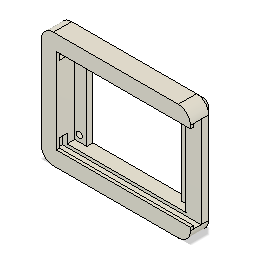
Displaygehäuse (Autodesk Fusion 360 design; units mm, degrees)
Autodesk Fusion 360 part; units mm, degrees
sketch "Skizze1" plane through (0, 0, 0) normal (0, 0, 1) x (1, 0, 0)
  line L0 (19.5, 14) -> (-19.5, 14)
  line L1 (-19.5, 14) -> (-19.5, -14)
  line L2 (-19.5, -14) -> (19.5, -14)
  line L3 (19.5, -14) -> (19.5, 14)
  line L4 (19.5, 14) -> (-19.5, -14) construction
  line L5 (-19.5, 14) -> (19.5, -14) construction
  line L6 (22.5, 17) -> (-22.5, 17)
  line L7 (-22.5, 17) -> (-22.5, -17)
  line L8 (-22.5, -17) -> (22.5, -17)
  line L9 (22.5, -17) -> (22.5, 17)
  line L10 (22.5, 17) -> (-22.5, -17) construction
  line L11 (-22.5, 17) -> (22.5, -17) construction
  line L12 (15.5, 14) -> (-15.5, 14)
  line L13 (-15.5, 14) -> (-15.5, -14)
  line L14 (-15.5, -14) -> (15.5, -14)
  line L15 (15.5, -14) -> (15.5, 14)
  line L16 (15.5, 14) -> (-15.5, -14) construction
  line L17 (-15.5, 14) -> (15.5, -14) construction
  line L18 (-19.5, 14) -> (-18.5, 14)
  circle A0 centre (-18, 12) radius 1
  circle A1 centre (-18, -12) radius 1
  circle A2 centre (18, -12) radius 1
  circle A3 centre (18, 12) radius 1
  dimension "d1" = 39
  dimension "d2" = 28
  dimension "d3" = 45
  dimension "d4" = 34
  dimension "d5" = 31
  dimension "d7" = 2
  dimension "d8" = 2
  dimension "d9" = 2
  dimension "d10" = 2
  constraint horizontal L0
  constraint perpendicular L0 L1
  constraint parallel L0 L2
  constraint parallel L1 L3
  constraint coincident L4 origin
  constraint coincident L5 origin
  constraint horizontal L6
  constraint perpendicular L6 L7
  constraint parallel L6 L8
  constraint parallel L7 L9
  constraint coincident L10 origin
  constraint coincident L11 origin
  constraint horizontal L12
  constraint perpendicular L12 L13
  constraint parallel L12 L14
  constraint parallel L13 L15
  constraint coincident L16 origin
  constraint coincident L17 origin
  constraint coincident L0 L18.end
  measures "d1" distance of L1.end L2.end
  measures "d2" distance of L0.end L1.end
  measures "d3" distance of L7.end L8.end
  measures "d4" distance of L6.start L8.end
  measures "d5" distance of L13.end L14.end
  measures "d7" diameter of A1
  measures "d8" diameter of A0
  measures "d9" diameter of A2
  measures "d10" diameter of A3
extrude "Extrusion1" add sketch "Skizze1" along normal blind 6 contours L6 L7 L8 L9
extrude "Extrusion2" add sketch "Skizze1" along normal blind 2 contours L0 L2 L3 L15 | L0 L1 L2 L13 L18
extrude "Extrusion3" add 1 faces at (-6.5, -16, 6) along direction (0, 0, 1) blind 2
extrude "Extrusion4" add 1 faces at (-22.5, -5.6667, 5.3333) along direction (-1, 0, 0) blind 2
extrude "Extrusion5" add 1 faces at (22.5, -5.6667, 2.6667) along direction (1, 0, 0) blind 2
extrude "Extrusion6" add 1 faces at (-8.1667, -17, 5.3333) along direction (0, -1, 0) blind 2
extrude "Extrusion7" add 1 faces at (8.1667, 17, 5.3333) along direction (0, 1, 0) blind 2
fillet "Abrundung1" radius 4 1 edges at (24.5, 19, 4)
fillet "Abrundung2" radius 4 1 edges at (-24.5, 19, 4)
fillet "Abrundung3" radius 4 1 edges at (-24.5, -19, 4)
fillet "Abrundung4" radius 4 1 edges at (24.5, -19, 4)
chamfer "Fase1" distance 2 angle 45 8 edges at (24.5, 0, 0) (23.3284, -17.8284, 0) (0, -19, 0) (-23.3284, -17.8284, 0) (-24.5, 0, 0) (-23.3284, 17.8284, 0) (0, 19, 0) (23.3284, 17.8284, 0)
sketch "Skizze2" plane through (24.5, 0, 0) normal (1, 0, 0) x (0, 0, -1)
  line L0 (-2, -15) -> (-2, 15)
  line L1 (-2, 15) -> (-8, 15)
  line L2 (-8, 15) -> (-8, -15)
  line L3 (-8, -15) -> (-2, -15)
  line L4 (-7, 15) -> (-4.5, 15)
  line L5 (-4.5, 15) -> (-4.5, -15)
  line L6 (-4.5, -15) -> (-7, -15)
  line L7 (-7, -15) -> (-7, 15)
  constraint horizontal L4
  constraint vertical L5
  constraint horizontal L6
  constraint vertical L7
  constraint coincident L3 L5.end
  constraint coincident L1 L4.start
extrude "Extrusion8" cut sketch "Skizze2" against normal blind 44 contours L1 L3 L4 L5 L6 L7
sketch "Skizze3" plane through (0, 0, 0) normal (1, 0, 0) x (0, 0, -1)
  line L0 (-4.5, -14) -> (-2, -14)
  line L1 (-2, -14) -> (-2, 14)
  line L2 (-2, 14) -> (-4.5, 14)
  line L3 (-4.5, 14) -> (-4.5, 15)
  line L4 (-4.5, 15) -> (-7, 15)
  line L5 (-7, 15) -> (-7, 14)
  line L6 (-7, 14) -> (-8, 14)
  line L7 (-8, 14) -> (-8, -14)
  line L8 (-8, -14) -> (-7, -14)
  line L9 (-7, -14) -> (-7, -15)
  line L10 (-7, -15) -> (-4.5, -15)
  line L11 (-4.5, -15) -> (-4.5, -14)
  line L12 (-7, 15) -> (-4.5, 15)
  line L13 (-4.5, 15) -> (-4.5, 11)
  line L14 (-4.5, 11) -> (-7, 11)
  line L15 (-7, 11) -> (-7, 15)
  line L16 (-7, -15) -> (-4.5, -15)
  line L17 (-4.5, -15) -> (-4.5, -11)
  line L18 (-4.5, -11) -> (-7, -11)
  line L19 (-7, -11) -> (-7, -15)
  dimension "d37" = 4
  dimension "d38" = 2.5
  dimension "d39" = 4
  dimension "d40" = 2.5
  constraint horizontal L12
  constraint vertical L13
  constraint horizontal L14
  constraint vertical L15
  constraint coincident L4.end L5.start
  constraint horizontal L16
  constraint vertical L17
  constraint horizontal L18
  constraint vertical L19
  constraint coincident L9.end L10.start
  measures "d37" distance of L4.end L14.end
  measures "d38" distance of L4.end L3.end
  measures "d39" distance of L9.end L18.end
  measures "d40" distance of L9.end L10.end
extrude "Extrusion9" cut sketch "Skizze3" against normal blind 21 contours L9 L10 L11 L16 L17 L18 L19 | L3 L4 L5 L12 L13 L14 L15
sketch "Skizze4" plane through (19.5, 0, 0) normal (-1, 0, 0) x (0, 0, 1)
  line L0 (7, 14) -> (7, -14)
  line L1 (7, -14) -> (8, -14)
  line L2 (8, -14) -> (8, 14)
  line L3 (8, 14) -> (7, 14)
  line L4 (7, 14) -> (8, 14)
  line L5 (8, 14) -> (8, -14)
  line L6 (8, -14) -> (7, -14)
  line L7 (7, -14) -> (7, 14)
  constraint horizontal L4
  constraint vertical L5
  constraint horizontal L6
  constraint vertical L7
  constraint coincident L1.end L2.start
  constraint coincident L0.start L3.end
extrude "Extrusion10" cut sketch "Skizze4" against normal blind 5
